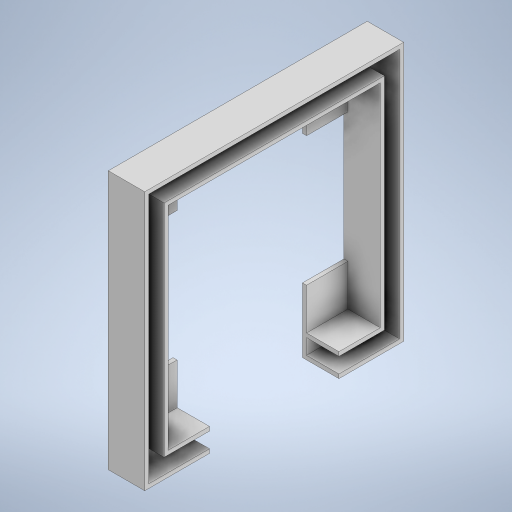
# Autodesk Inventor part: end cap
Saved by Autodesk Inventor 2024 (Build 280153000, 153)
## iProperties
Created: 2024-08-01
Part Number: end cap
Material: Generic
Document SubType Name: Modeling
Designer: kherron1
Density: 1 g/cm^3
Appearance: Default
Author: kherron1
Autodesk Inventor part; units mm, degrees
ref_plane "YZ Plane" through (0, 0, 0) normal (1, 0, 0) x (0, 1, 0)
ref_plane "XZ Plane" through (0, 0, 0) normal (0, 1, 0) x (-1, 0, 0)
ref_plane "XY Plane" through (0, 0, 0) normal (0, 0, 1) x (1, 0, 0)
sketch "Sketch3" plane through (0, 0, 0) normal (1, 0, 0) x (0, 1, 0)
  line L0 (0, 0) -> (25.4, 0)
  line L1 (25.4, 0) -> (25.4, -25.4)
  line L2 (25.4, -25.4) -> (0, -25.4)
  line L3 (0, -25.4) -> (0, 0)
  line L4 (25.4, -23.8125) -> (1.5875, -23.8125)
  line L5 (1.5875, -23.8125) -> (1.5875, 0)
  line L6 (7.5819, -17.8125) -> (25.4, -17.8125)
  line L7 (7.5819, 0) -> (7.5819, -17.8125)
  line L8 (9.1694, 1) -> (9.1694, -16.225)
  line L9 (9.1694, -16.225) -> (25.4, -16.225)
  point P0 (25.4, -16.225)
  point P1 (9.1694, 0)
  dimension "d15" = 25.4
  dimension "d16" = 25.4
  dimension "d17" = 1.5875
  dimension "d18" = 6
  dimension "d19" = 1.5875
  dimension "d24" = 5.9944
  constraints: 20 end point, 4 point on line, 2 parallel, 1 horizontal, 1 perpendicular, 1 other
  measures "d15" distance of L1.end L2.end
  measures "d16" distance of L0.end L1.end
  measures "d17" distance between parallel lines of L3 L5
  measures "d18" distance between parallel lines of L4 L6
  measures "d19" distance between parallel lines of L7 L8
  measures "d24" distance between parallel lines of L5 L7
extrude "Extrusion3" add sketch "Sketch3" along normal blind 25.4 contours L0 L5 L4 L1 L2 L3 | L0 L8 L9 L1 L6 L7
sketch "Sketch4" plane through (0, 0, 0) normal (-1, 0, 0) x (0, 0, 1)
  line L0 (-25.4, 0) -> (-25.4, 25.4) projected
  line L1 (-25.4, 25.4) -> (0, 25.4)
  line L2 (0, 25.4) -> (0, 0)
  line L3 (0, 0) -> (-25.4, 0)
  line L4 (-25.4, 0) -> (-25.4, 25.4)
  constraints: 8 end point, 2 parallel, 1 horizontal, 1 perpendicular
extrude "Extrusion4" add sketch "Sketch4" along normal blind 1.5875
sketch "Sketch5" plane through (25.4, 7.5819, 0) normal (0, 0, 1) x (1, 0, 0)
  line L0 (-25.4, 0) -> (0, 0) projected
  line L1 (0, 1.5875) -> (0, 0) projected
  line L2 (-25.4, 1.5875) -> (0, 1.5875) projected
  line L3 (-25.4, 1.5875) -> (-25.4, 17.8181) projected
  line L4 (-25.4, 17.8181) -> (-26.9875, 17.8181) projected
  line L5 (-26.9875, -7.5819) -> (-26.9875, 17.8181) projected
  line L6 (-26.9875, -7.5819) -> (0, -7.5819) projected
  line L7 (0, -5.9944) -> (0, -7.5819) projected
  line L8 (-25.4, -5.9944) -> (0, -5.9944) projected
  line L9 (-25.4, -5.9944) -> (-25.4, 0) projected
  line L10 (-26.9875, 1.5875) -> (-25.4, 1.5875)
  point P0 (-25.4, -7.5819)
  constraints: 2 end point, 1 collinear, 1 point on line
extrude "Extrusion5" add sketch "Sketch5" along normal blind 25.4 contours L9 L8 L7 L6 L5 L10 L2 L1 L0
sketch "Sketch6" plane through (25.4, 25.4, -16.225) normal (0, 1, 0) x (1, 0, 0)
  line L0 (-25.4, 0) -> (0, 0) projected
  line L1 (0, 1.5875) -> (0, 0) projected
  line L2 (-25.4, 1.5875) -> (0, 1.5875) projected
  line L3 (-25.4, 1.5875) -> (-25.4, 7.5875) projected
  line L4 (-25.4, 7.5875) -> (0, 7.5875) projected
  line L5 (0, 9.175) -> (0, 7.5875) projected
  line L6 (-26.9875, 9.175) -> (0, 9.175) projected
  line L7 (-26.9875, -16.225) -> (-26.9875, 9.175) projected
  line L8 (-25.4, -16.225) -> (-26.9875, -16.225) projected
  line L9 (-25.4, -16.225) -> (-25.4, 0) projected
  line L10 (-26.9875, 0) -> (-25.4, 0)
  point P0 (-25.4, -16.225)
  constraints: 2 end point, 1 horizontal, 1 point on line
extrude "Extrusion6" add sketch "Sketch6" along normal blind 25.4 contours L10 L7 L6 L5 L4 L3 L2 L1 L0
mirror "Mirror1" about plane through (11.9062, 4.5847, 25.4) normal (0, 0, 1)
mirror "Mirror2" about plane through (11.9062, 50.8, -20.8125) normal (0, 1, 0)
sketch "Sketch7" plane through (-1.5875, 0, 76.2) normal (0, 0, 1) x (1, 0, 0)
  line L0 (26.9875, 0) -> (0, 0) projected
  line L1 (26.9875, 0) -> (14.2875, 0)
  line L2 (14.2875, 0) -> (14.2875, 107.076)
  line L3 (14.2875, 107.076) -> (26.9875, 107.076)
  line L4 (26.9875, 107.076) -> (26.9875, 0)
  point P0 (1.5875, 0)
  dimension "d29" = 12.7
  constraints: 8 end point, 2 parallel, 1 horizontal, 1 perpendicular
  measures "d29" distance of L2.end L3.end
extrude "Extrusion7" cut sketch "Sketch7" against normal blind 161.925
sketch "Sketch8" plane through (-1.5875, 0, 0) normal (-1, 0, 0) x (0, 0, 1)
  line L0 (0, 9.1694) -> (50.8, 9.1694) projected
  line L1 (0, 9.1694) -> (50.8, 9.1694)
  line L2 (50.8, 9.1694) -> (50.8, -7.9488)
  line L3 (50.8, -7.9488) -> (0, -7.9488)
  line L4 (0, -7.9488) -> (0, 9.1694)
  point P0 (0, 0)
  constraints: 8 end point, 2 parallel, 1 horizontal, 1 perpendicular
extrude "Extrusion8" cut sketch "Sketch8" against normal blind 161.925
body "Solid2"
